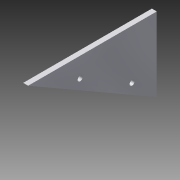
# Autodesk Inventor part: 30deg gusset plate
Saved by Autodesk Inventor 2015 SP1 (Build 190203100, 203)
## iProperties
Created: 2015-01-30
Part Number: 30deg gusset plate
Material: Generic
Document SubType Name: Modeling
Designer: Admin
Density: 1 g/cm^3
Appearance: Default
Author: Admin
Autodesk Inventor part; units mm, degrees
ref_plane "YZ Plane" through (0, 0, 0) normal (1, 0, 0) x (0, 1, 0)
ref_plane "XZ Plane" through (0, 0, 0) normal (0, 1, 0) x (-1, 0, 0)
ref_plane "XY Plane" through (0, 0, 0) normal (0, 0, 1) x (1, 0, 0)
sketch "Sketch1" plane through (0, 0, 0) normal (1, 0, 0) x (0, 1, 0)
  line L0 (0, 0) -> (0, 165.1)
  line L1 (0, 0) -> (-95.25, 0)
  line L2 (-95.25, 0) -> (0, 165.1)
  dimension "d0" = 165.1
  dimension "d1" = 95.25
  constraints: 6 end point, 1 horizontal, 1 vertical
  measures "d0" distance of L0.start L0.end
  measures "d1" distance of L0.start L1.end
extrude "Extrusion1" add sketch "Sketch1" along normal blind 6.35
sketch "Sketch2" plane through (0, 0, 0) normal (-1, 0, 0) x (0, 0, 1)
  line L0 (0, 0) -> (165.1, 0) projected
  line L1 (0, -95.25) -> (0, 0) projected
  point P0 (98.425, -25.4)
  point P1 (31.75, -63.5)
  dimension "d4" = 25.4
  dimension "d5" = 98.425
  dimension "d6" = 31.75
  dimension "d7" = 63.5
  measures "d4" distance from line of point (98.425, -25.4) L0
  measures "d5" distance from line of L1 point (98.425, -25.4)
  measures "d6" distance from line of L1 point (31.75, -63.5)
  measures "d7" distance from line of L0 point (31.75, -63.5)
hole "Hole1" at (0, -25.4, 98.425) at (0, -63.5, 31.75) direction (1, 0, 0) diameter 6.35 end through all
body "Solid1"
